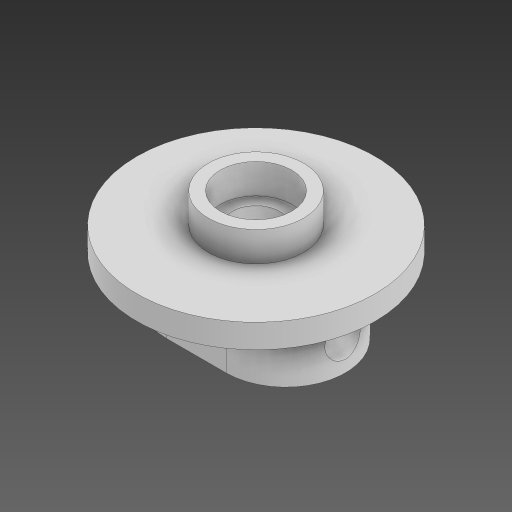
# Autodesk Inventor part: koleso_rig
Saved by Autodesk Inventor 2023 (Build 270158000, 158)
## iProperties
Created: 2025-05-29
Part Number: koleso_rig
Material: Типовые
Document SubType Name: Modeling
Designer: daa
Density: 1 g/cm^3
Appearance: По умолчанию
Author: daa
Autodesk Inventor part; units mm, degrees
ref_plane "YZ Plane" through (0, 0, 0) normal (1, 0, 0) x (0, 1, 0)
ref_plane "XZ Plane" through (0, 0, 0) normal (0, 1, 0) x (-1, 0, 0)
ref_plane "XY Plane" through (0, 0, 0) normal (0, 0, 1) x (1, 0, 0)
sketch "Эскиз1" plane through (0, 0, 0) normal (0, 1, 0) x (-1, 0, 0)
  circle A0 centre (0, 0) radius 10
  dimension "d0" = 20
  constraints: 1 centre point, 1 coincident
  measures "d0" diameter of A0
extrude "Выдавливание1" add sketch "Эскиз1" along normal blind 2
sketch "Эскиз2" plane through (0, 2, 0) normal (0, 1, 0) x (1, 0, 0)
  circle A0 centre (0, 0) radius 4
  circle A1 centre (0, 0) radius 3
  dimension "d3" = 8
  dimension "d4" = 6
  constraints: 2 centre point, 2 coincident
  measures "d3" diameter of A0
  measures "d4" diameter of A1
extrude "Выдавливание2" add sketch "Эскиз2" along normal blind 2.5
sketch "Эскиз3" plane through (0, 0, 0) normal (0, -1, 0) x (1, 0, 0)
  line L0 (7.5, -5) -> (-7.5, -5)
  line L1 (-7.5, -5) -> (-7.5, 5)
  line L2 (-7.5, 5) -> (7.5, 5)
  line L3 (7.5, 5) -> (7.5, -5)
  line L4 (5, -2.85) -> (2.4, -2.85)
  line L5 (2.4, -2.85) -> (2.4, 2.85)
  line L6 (2.4, 2.85) -> (5, 2.85)
  line L7 (5, 2.85) -> (5, -2.85)
  line L8 (-2.4, -2.85) -> (-5, -2.85)
  line L9 (-5, -2.85) -> (-5, 2.85)
  line L10 (-5, 2.85) -> (-2.4, 2.85)
  line L11 (-2.4, 2.85) -> (-2.4, -2.85)
  circle A0 centre (0, 0) radius 2
  dimension "d7" = 15
  dimension "d8" = 10
  dimension "d9" = 7.5
  dimension "d10" = 5
  dimension "d11" = 2.6
  dimension "d12" = 5.7
  dimension "d13" = 2.6
  dimension "d14" = 5.7
  dimension "d15" = 2.15
  dimension "d16" = 2.15
  dimension "d17" = 2.5
  dimension "d18" = 2.5
  dimension "d19" = 4
  constraints: 24 end point, 6 parallel, 3 horizontal, 3 perpendicular, 1 centre point, 1 coincident
  measures "d7" distance of L1.end L2.end
  measures "d8" distance of L0.end L1.end
  measures "d9" distance from line of L1 point (0, 0)
  measures "d10" distance from line of point (0, 0) L0
  measures "d11" distance of L5.end L6.end
  measures "d12" distance of L4.end L5.end
  measures "d13" distance of L9.end L10.end
  measures "d14" distance of L8.end L9.end
  measures "d15" distance between parallel lines of L2 L6
  measures "d16" distance between parallel lines of L2 L10
  measures "d17" distance between parallel lines of L1 L9
  measures "d18" distance between parallel lines of L7 L3
  measures "d19" diameter of A0
extrude "Выдавливание3" add sketch "Эскиз3" along normal blind 5
sketch "Эскиз4" plane through (7.5, 0, 5) normal (1, 0, 0) x (0, 0, -1)
  circle A0 centre (5, -2.5) radius 1.5
  line L0 (10, -5) -> (0, -5) projected
  line L1 (0, 0) -> (0, -5) projected
  point P0 (5, 0)
  point P1 (0, -2.5)
  dimension "d22" = 3
  dimension "d23" = 2.5
  dimension "d24" = 5
  constraints: 1 centre point, 1 midpoint
  measures "d22" diameter of A0
  measures "d23" distance from line of L0 A0.centre
  measures "d24" distance of point (0, -2.5) A0.centre
extrude "Выдавливание4" cut sketch "Эскиз4" against normal blind 22.5
fillet "Сопряжение1" radius 5 4 edges at (7.5, -2.5, -5) (7.5, -2.5, 5) (-7.5, -2.5, 5) (-7.5, -2.5, -5)
sketch "Эскиз5" plane through (0, 2, 0) normal (0, 1, 0) x (1, 0, 0)
  circle A0 centre (0, 0) radius 2
  dimension "d28" = 4
  constraints: 1 centre point, 1 coincident
  measures "d28" diameter of A0
extrude "Выдавливание5" cut sketch "Эскиз5" against normal blind 11
